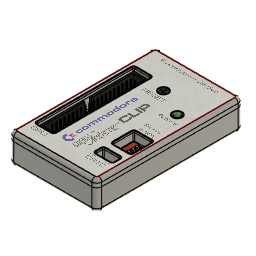
PETDiag_Clip_v3 v11 (Autodesk Fusion 360 design; units mm, degrees)
Autodesk Fusion 360 part; units mm, degrees
(part 1 of 3)
sketch "dxf" plane through (0, 0, 0) normal (0, 0, 1) x (1, 0, 0) in component "PCB"
  line L0 (47, 0) -> (47, 77)
  line L1 (0, 77) -> (0, 0)
  line L2 (0, 0) -> (47, 0)
  line L3 (47, 77) -> (0, 77)
  line L4 (1.7462, 63.1975) -> (1.7462, 63.3563)
  arc A0 (16.383, 5.334) -> (16.383, 7.366) centre (16.383, 6.35) ccw
  arc A1 (23.3363, 18.542) -> (20.7963, 18.542) centre (22.0663, 18.542) ccw
  circle A2 centre (5, 72) radius 3.1789
  line L5 (1.7462, 63.3563) -> (1.7462, 63.515)
  line L6 (1.7462, 40.8138) -> (1.7462, 62.0863)
  line L7 (1.7462, 63.6738) -> (1.7462, 67.96)
  line L8 (28.6703, 53.848) -> (15.4623, 53.848)
  line L9 (1.7462, 62.0863) -> (1.7462, 62.4038)
  line L10 (8.0963, 67.96) -> (9.525, 67.96)
  line L11 (1.7462, 63.515) -> (1.7462, 63.6738)
  line L12 (10.9538, 9.54) -> (9.525, 9.54)
  line L13 (23.3362, 18.542) -> (28.6703, 18.542)
  circle A3 centre (5, 5) radius 3.1789
  line L14 (15.4623, 18.542) -> (15.4623, 53.848)
  line L15 (1.7462, 67.96) -> (8.0963, 67.96)
  line L16 (16.383, 3.302) -> (35.687, 3.302)
  line L17 (1.7462, 62.88) -> (1.7462, 63.0388)
  line L18 (9.525, 9.54) -> (8.0963, 9.54)
  line L19 (1.7462, 62.7213) -> (1.7462, 62.88)
  line L20 (35.687, 9.398) -> (16.383, 9.398)
  line L21 (8.0963, 10.3337) -> (8.0963, 9.54)
  line L22 (2.54, 40.8138) -> (1.7462, 40.8138)
  line L23 (10.16, 67.1663) -> (10.16, 10.3337)
  line L24 (1.7462, 9.54) -> (1.7462, 36.6862)
  line L25 (3.0162, 10.81) -> (2.54, 10.3337)
  line L26 (28.6703, 18.542) -> (28.6703, 53.848)
  line L27 (7.366, 62.626) -> (7.874, 62.626)
  line L28 (8.0963, 10.3337) -> (2.54, 10.3337)
  line L29 (9.525, 66.69) -> (9.6838, 66.69)
  line L30 (9.525, 10.81) -> (8.0963, 10.81)
  line L31 (3.0162, 40.8138) -> (3.0162, 66.69)
  line L32 (1.7462, 36.6862) -> (1.7462, 40.8138)
  line L33 (8.0963, 66.69) -> (8.0963, 67.1663)
  arc A4 (10.9538, 38.2738) -> (10.9538, 39.385) centre (10.9538, 38.8294) ccw
  line L34 (15.4623, 18.542) -> (20.7963, 18.542)
  line L35 (1.7462, 62.5625) -> (1.7462, 62.7213)
  line L36 (1.7462, 63.1975) -> (1.7462, 63.0388)
  line L37 (2.54, 36.6862) -> (1.7462, 36.6862)
  line L38 (9.6838, 10.81) -> (9.525, 10.81)
  line L39 (8.0963, 9.54) -> (1.7462, 9.54)
  line L40 (3.0162, 36.6862) -> (2.54, 36.6862)
  line L41 (9.6838, 66.69) -> (9.6838, 10.81)
  line L42 (3.0162, 10.81) -> (3.0162, 36.6862)
  line L43 (1.7462, 62.5625) -> (1.7463, 62.5625)
  line L44 (8.0963, 10.81) -> (3.0162, 10.81)
  circle A5 centre (5, 5) radius 1.7463
  circle A6 centre (42, 72) radius 1.7463
  line L45 (35.687, 9.398) -> (35.687, 3.302)
  line L46 (9.525, 10.3337) -> (10.16, 10.3337)
  line L47 (16.383, 9.398) -> (16.383, 7.366)
  circle A7 centre (42, 5) radius 1.7463
  line L48 (4.826, 62.626) -> (5.334, 62.626)
  line L49 (9.525, 10.81) -> (9.525, 10.3337)
  line L50 (9.525, 66.69) -> (9.525, 67.1663)
  line L51 (16.383, 3.302) -> (16.383, 5.334)
  arc A8 (10.9538, 65.42) -> (10.9538, 66.69) centre (10.9538, 66.055) ccw
  line L52 (8.0963, 67.1663) -> (8.0963, 67.96)
  line L53 (9.525, 10.3337) -> (9.525, 9.54)
  line L54 (5.334, 62.626) -> (5.334, 63.134)
  line L55 (9.525, 67.1663) -> (9.525, 67.96)
  line L56 (3.0162, 66.69) -> (8.0963, 66.69)
  line L57 (10.16, 67.1663) -> (9.6838, 66.69)
  line L58 (1.7462, 62.4038) -> (1.7462, 62.5625)
  line L59 (10.9538, 67.96) -> (10.9538, 9.54)
  circle A9 centre (5, 72) radius 1.7463
  line L60 (2.2225, 62.7213) -> (2.2224, 62.7213)
  line L61 (10.16, 67.1663) -> (9.525, 67.1663)
  circle A10 centre (42, 72) radius 3.1789
  line L62 (2.54, 62.88) -> (2.5399, 62.88)
  line L63 (8.0963, 67.1663) -> (2.54, 67.1663)
  circle A11 centre (42, 5) radius 3.1789
  line L64 (5.334, 55.006) -> (5.334, 55.514)
  line L65 (7.366, 57.546) -> (7.874, 57.546)
  line L66 (7.366, 52.974) -> (7.366, 52.466)
  line L67 (7.874, 52.466) -> (7.874, 52.974)
  line L68 (4.826, 58.054) -> (4.826, 57.546)
  line L69 (5.334, 55.514) -> (4.826, 55.514)
  line L70 (5.334, 60.086) -> (5.334, 60.594)
  line L71 (4.826, 57.546) -> (5.334, 57.546)
  line L72 (7.874, 60.594) -> (7.366, 60.594)
  line L73 (4.826, 63.134) -> (4.826, 62.626)
  line L74 (7.874, 63.134) -> (7.366, 63.134)
  line L75 (7.366, 52.466) -> (7.874, 52.466)
  line L76 (7.874, 55.514) -> (7.366, 55.514)
  line L77 (4.826, 55.514) -> (4.826, 55.006)
  line L78 (4.826, 60.086) -> (5.334, 60.086)
  line L79 (2.54, 36.6862) -> (2.54, 10.3337)
  line L80 (4.826, 49.926) -> (5.334, 49.926)
  line L81 (7.874, 49.926) -> (7.874, 50.434)
  line L82 (4.826, 52.466) -> (5.334, 52.466)
  line L83 (7.366, 58.054) -> (7.366, 57.546)
  line L84 (7.874, 52.974) -> (7.366, 52.974)
  line L85 (3.0162, 36.6862) -> (3.0162, 40.8138)
  line L86 (9.6838, 10.81) -> (10.16, 10.3337)
  line L87 (5.334, 47.894) -> (4.826, 47.894)
  line L88 (7.366, 49.926) -> (7.874, 49.926)
  line L89 (9.525, 67.96) -> (10.9538, 67.96)
  line L90 (2.54, 62.88) -> (2.54, 67.1663)
  line L91 (7.366, 50.434) -> (7.366, 49.926)
  line L92 (5.334, 52.974) -> (4.826, 52.974)
  line L93 (7.366, 44.846) -> (7.874, 44.846)
  line L94 (7.874, 57.546) -> (7.874, 58.054)
  line L95 (2.54, 40.8138) -> (2.54, 62.88)
  line L96 (4.826, 60.594) -> (4.826, 60.086)
  line L97 (7.874, 55.006) -> (7.874, 55.514)
  line L98 (7.366, 55.514) -> (7.366, 55.006)
  line L99 (4.826, 50.434) -> (4.826, 49.926)
  line L100 (7.874, 50.434) -> (7.366, 50.434)
  line L101 (5.334, 50.434) -> (4.826, 50.434)
  line L102 (5.334, 58.054) -> (4.826, 58.054)
  line L103 (7.366, 45.354) -> (7.366, 44.846)
  arc A12 (10.9538, 10.81) -> (10.9538, 12.08) centre (10.9538, 11.445) ccw
  line L104 (5.334, 49.926) -> (5.334, 50.434)
  line L105 (4.826, 47.386) -> (5.334, 47.386)
  line L106 (5.334, 47.386) -> (5.334, 47.894)
  line L107 (4.826, 55.006) -> (5.334, 55.006)
  line L108 (7.366, 60.594) -> (7.366, 60.086)
  line L109 (3.0162, 40.8138) -> (2.54, 40.8138)
  line L110 (5.334, 63.134) -> (4.826, 63.134)
  line L111 (8.0963, 10.81) -> (8.0963, 10.3337)
  line L112 (7.874, 62.626) -> (7.874, 63.134)
  line L113 (2.54, 67.1663) -> (3.0162, 66.69)
  line L114 (8.0963, 66.69) -> (9.525, 66.69)
  line L115 (7.874, 60.086) -> (7.874, 60.594)
  line L116 (7.366, 63.134) -> (7.366, 62.626)
  line L117 (7.366, 47.386) -> (7.874, 47.386)
  line L118 (5.334, 60.594) -> (4.826, 60.594)
  line L119 (5.334, 52.466) -> (5.334, 52.974)
  line L120 (7.874, 47.894) -> (7.366, 47.894)
  line L121 (7.874, 47.386) -> (7.874, 47.894)
  line L122 (4.826, 47.894) -> (4.826, 47.386)
  line L123 (7.874, 58.054) -> (7.366, 58.054)
  line L124 (7.366, 34.686) -> (7.874, 34.686)
  line L125 (7.366, 32.654) -> (7.366, 32.146)
  line L126 (4.826, 32.654) -> (4.826, 32.146)
  line L127 (7.874, 32.654) -> (7.366, 32.654)
  line L128 (7.366, 47.894) -> (7.366, 47.386)
  line L129 (7.366, 37.734) -> (7.366, 37.226)
  line L130 (4.826, 39.766) -> (5.334, 39.766)
  line L131 (5.334, 45.354) -> (4.826, 45.354)
  line L132 (7.874, 40.274) -> (7.366, 40.274)
  line L133 (7.874, 30.114) -> (7.366, 30.114)
  line L134 (7.874, 42.306) -> (7.874, 42.814)
  line L135 (7.366, 60.086) -> (7.874, 60.086)
  line L136 (7.874, 42.814) -> (7.366, 42.814)
  line L137 (5.334, 32.654) -> (4.826, 32.654)
  line L138 (5.334, 37.734) -> (4.826, 37.734)
  line L139 (5.334, 42.814) -> (4.826, 42.814)
  line L140 (5.334, 40.274) -> (4.826, 40.274)
  line L141 (7.366, 55.006) -> (7.874, 55.006)
  line L142 (4.826, 42.814) -> (4.826, 42.306)
  line L143 (5.334, 42.306) -> (5.334, 42.814)
  line L144 (7.874, 44.846) -> (7.874, 45.354)
  line L145 (7.874, 32.146) -> (7.874, 32.654)
  line L146 (7.874, 45.354) -> (7.366, 45.354)
  line L147 (7.874, 34.686) -> (7.874, 35.194)
  line L148 (5.334, 39.766) -> (5.334, 40.274)
  line L149 (4.826, 44.846) -> (5.334, 44.846)
  line L150 (7.366, 35.194) -> (7.366, 34.686)
  line L151 (4.826, 40.274) -> (4.826, 39.766)
  line L152 (7.366, 32.146) -> (7.874, 32.146)
  line L153 (5.334, 25.034) -> (4.826, 25.034)
  line L154 (4.826, 19.446) -> (5.334, 19.446)
  line L155 (4.826, 32.146) -> (5.334, 32.146)
  line L156 (5.334, 29.606) -> (5.334, 30.114)
  line L157 (5.334, 19.954) -> (4.826, 19.954)
  line L158 (4.826, 25.034) -> (4.826, 24.526)
  line L159 (4.826, 34.686) -> (5.334, 34.686)
  line L160 (4.826, 35.194) -> (4.826, 34.686)
  line L161 (4.826, 37.226) -> (5.334, 37.226)
  line L162 (7.874, 37.226) -> (7.874, 37.734)
  line L163 (4.826, 45.354) -> (4.826, 44.846)
  line L164 (7.874, 29.606) -> (7.874, 30.114)
  line L165 (7.366, 37.226) -> (7.874, 37.226)
  line L166 (7.366, 42.306) -> (7.874, 42.306)
  line L167 (7.874, 39.766) -> (7.874, 40.274)
  line L168 (7.366, 29.606) -> (7.874, 29.606)
  line L169 (5.334, 37.226) -> (5.334, 37.734)
  line L170 (7.366, 40.274) -> (7.366, 39.766)
  line L171 (4.826, 19.954) -> (4.826, 19.446)
  line L172 (4.826, 21.986) -> (5.334, 21.986)
  line L173 (7.366, 30.114) -> (7.366, 29.606)
  line L174 (5.334, 27.574) -> (4.826, 27.574)
  line L175 (5.334, 57.546) -> (5.334, 58.054)
  line L176 (4.826, 52.974) -> (4.826, 52.466)
  line L177 (5.334, 32.146) -> (5.334, 32.654)
  line L178 (7.874, 35.194) -> (7.366, 35.194)
  line L179 (5.334, 44.846) -> (5.334, 45.354)
  line L180 (7.366, 39.766) -> (7.874, 39.766)
  line L181 (7.366, 42.814) -> (7.366, 42.306)
  line L182 (4.826, 37.734) -> (4.826, 37.226)
  line L183 (7.874, 37.734) -> (7.366, 37.734)
  line L184 (4.826, 30.114) -> (4.826, 29.606)
  line L185 (5.334, 34.686) -> (5.334, 35.194)
  line L186 (4.826, 42.306) -> (5.334, 42.306)
  line L187 (5.334, 35.194) -> (4.826, 35.194)
  line L188 (5.334, 22.494) -> (4.826, 22.494)
  line L189 (34.29, 53.975) -> (33.02, 53.975)
  line L190 (28.2575, 15.7163) -> (28.2575, 11.9063)
  line L191 (34.29, 48.895) -> (33.02, 48.895)
  line L192 (25.0825, 11.2713) -> (25.7175, 11.9063)
  line L193 (30.7975, 15.7163) -> (30.7975, 11.9063)
  line L194 (7.874, 19.954) -> (7.366, 19.954)
  line L195 (5.334, 21.986) -> (5.334, 22.494)
  line L196 (23.8125, 16.3513) -> (25.0825, 16.3513)
  line L197 (7.366, 25.034) -> (7.366, 24.526)
  line L198 (5.334, 19.446) -> (5.334, 19.954)
  line L199 (7.366, 16.906) -> (7.874, 16.906)
  line L200 (26.3525, 11.2713) -> (27.6225, 11.2713)
  line L201 (25.7175, 15.7163) -> (25.7175, 11.9063)
  line L202 (5.334, 16.906) -> (5.334, 17.414)
  line L203 (4.826, 17.414) -> (4.826, 16.906)
  line L204 (26.3525, 16.3513) -> (27.6225, 16.3513)
  line L205 (28.2575, 15.7163) -> (28.8925, 16.3513)
  line L206 (7.874, 24.526) -> (7.874, 25.034)
  line L207 (4.826, 14.874) -> (4.826, 14.366)
  line L208 (7.874, 19.446) -> (7.874, 19.954)
  line L209 (7.874, 25.034) -> (7.366, 25.034)
  line L210 (7.874, 27.066) -> (7.874, 27.574)
  line L211 (7.366, 27.574) -> (7.366, 27.066)
  line L212 (7.874, 27.574) -> (7.366, 27.574)
  line L213 (23.1775, 11.9063) -> (23.1775, 15.7163)
  line L214 (7.874, 14.874) -> (7.366, 14.874)
  line L215 (32.385, 52.07) -> (32.385, 53.975)
  line L216 (7.366, 19.446) -> (7.874, 19.446)
  line L217 (5.334, 30.114) -> (4.826, 30.114)
  line L218 (7.366, 19.954) -> (7.366, 19.446)
  line L219 (4.826, 16.906) -> (5.334, 16.906)
  line L220 (7.366, 21.986) -> (7.874, 21.986)
  line L221 (25.7175, 11.9063) -> (26.3525, 11.2713)
  line L222 (32.385, 49.53) -> (32.385, 50.8)
  line L223 (33.02, 53.975) -> (32.385, 53.975)
  line L224 (34.925, 50.8) -> (34.925, 49.53)
  line L225 (4.826, 22.494) -> (4.826, 21.986)
  line L226 (7.874, 14.366) -> (7.874, 14.874)
  line L227 (5.334, 14.366) -> (5.334, 14.874)
  line L228 (5.334, 27.066) -> (5.334, 27.574)
  line L229 (4.826, 27.066) -> (5.334, 27.066)
  line L230 (5.334, 14.874) -> (4.826, 14.874)
  line L231 (4.826, 27.574) -> (4.826, 27.066)
  line L232 (27.6225, 11.2713) -> (28.2575, 11.9063)
  line L233 (7.366, 14.874) -> (7.366, 14.366)
  line L234 (7.874, 17.414) -> (7.366, 17.414)
  line L235 (7.366, 22.494) -> (7.366, 21.986)
  line L236 (7.874, 22.494) -> (7.366, 22.494)
  line L237 (5.334, 17.414) -> (4.826, 17.414)
  line L238 (5.334, 24.526) -> (5.334, 25.034)
  line L239 (7.874, 21.986) -> (7.874, 22.494)
  line L240 (7.366, 24.526) -> (7.874, 24.526)
  line L241 (7.366, 27.066) -> (7.874, 27.066)
  line L242 (7.366, 17.414) -> (7.366, 16.906)
  line L243 (4.826, 24.526) -> (5.334, 24.526)
  line L244 (4.826, 14.366) -> (5.334, 14.366)
  line L245 (7.366, 14.366) -> (7.874, 14.366)
  line L246 (4.826, 29.606) -> (5.334, 29.606)
  line L247 (7.874, 16.906) -> (7.874, 17.414)
  line L248 (34.925, 52.07) -> (34.6075, 51.7525)
  line L249 (27.6225, 16.3513) -> (28.2575, 15.7163)
  line L250 (34.6075, 51.1175) -> (34.925, 50.8)
  line L251 (34.925, 53.34) -> (34.925, 52.07)
  circle A13 centre (23, 65) radius 1.75
  arc A14 (25.45, 63.25) -> (25.45, 62.45) centre (25.15, 62.85) ccw
  line L252 (34.925, 53.34) -> (34.29, 53.975)
  line L253 (25.7175, 15.7163) -> (26.3525, 16.3513)
  line L254 (32.7025, 51.7525) -> (32.385, 52.07)
  line L255 (30.1625, 11.2713) -> (30.7975, 11.9063)
  line L256 (45.7518, 33.9408) -> (42.4498, 33.9408)
  line L257 (26, 66.45) -> (26, 63.6)
  line L258 (23.1775, 11.9063) -> (23.1775, 11.2713)
  line L259 (30.1625, 16.3513) -> (30.7975, 15.7163)
  line L260 (25.0825, 16.3513) -> (25.7175, 15.7163)
  line L261 (28.8925, 16.3513) -> (30.1625, 16.3513)
  line L262 (32.385, 50.8) -> (32.7025, 51.1175)
  line L263 (23.1775, 11.2713) -> (25.0825, 11.2713)
  line L264 (28.8925, 11.2713) -> (30.1625, 11.2713)
  arc A15 (20.55, 62.45) -> (20.5, 63.2) centre (20.8502, 62.8467) ccw
  circle A16 centre (23, 65) radius 1.4
  line L265 (28.2575, 11.9063) -> (28.8925, 11.2713)
  line L266 (23.1775, 15.7163) -> (23.8125, 16.3513)
  line L267 (25.4, 62) -> (20.25, 62)
  line L268 (20, 63.55) -> (20, 66.45)
  arc A17 (20.55, 66.75) -> (20.5, 67.5) centre (20.8502, 67.1467) ccw
  line L269 (33.02, 48.895) -> (32.385, 49.53)
  line L270 (34.925, 49.53) -> (34.29, 48.895)
  line L271 (39.1478, 33.4327) -> (42.4498, 33.4327)
  line L272 (20.25, 68) -> (25.75, 68)
  line L273 (41.6878, 32.6707) -> (38.8938, 32.6707)
  line L274 (39.1478, 33.9408) -> (35.8458, 33.9408)
  line L275 (42.4498, 32.6707) -> (42.7037, 32.6707)
  line L276 (38.8938, 23.5267) -> (41.6878, 23.5267)
  line L277 (41.6878, 25.0508) -> (38.8938, 25.0508)
  line L278 (38.8938, 23.5267) -> (38.8938, 25.0508)
  line L279 (42.7037, 31.1468) -> (42.4498, 31.1468)
  line L280 (40.7988, 24.7968) -> (39.1478, 24.7968)
  line L281 (42.7037, 28.8608) -> (42.7037, 28.6068)
  line L282 (42.7037, 23.5267) -> (42.4498, 23.5267)
  line L283 (42.7037, 25.0508) -> (42.7037, 24.7968)
  line L284 (40.7988, 29.8768) -> (39.1478, 29.8768)
  line L285 (42.4498, 30.1308) -> (42.7037, 30.1308)
  line L286 (38.8938, 31.1468) -> (41.6878, 31.1468)
  line L287 (40.7988, 26.3208) -> (39.1478, 26.3208)
  line L288 (42.4498, 33.4327) -> (42.4498, 33.9408)
  line L289 (42.7037, 31.4008) -> (42.7037, 31.1468)
  line L290 (38.8938, 28.6068) -> (38.8938, 30.1308)
  line L291 (42.7037, 26.3208) -> (42.7037, 26.0668)
  line L292 (40.7988, 28.8608) -> (39.1478, 28.8608)
  line L293 (40.7988, 27.3368) -> (39.1478, 27.3368)
  line L294 (39.1478, 29.8768) -> (39.1478, 28.8608)
  line L295 (41.6878, 30.1308) -> (38.8938, 30.1308)
  line L296 (38.8938, 28.6068) -> (41.6878, 28.6068)
  line L297 (39.1478, 33.9408) -> (39.1478, 33.4327)
  line L298 (42.7037, 27.5907) -> (42.7037, 27.3368)
  line L299 (38.8938, 26.0668) -> (38.8938, 27.5907)
  line L300 (42.7037, 30.1308) -> (42.7037, 29.8768)
  arc A18 (25.45, 67.55) -> (25.5, 66.8) centre (25.1498, 67.1533) ccw
  line L301 (42.7037, 32.6707) -> (42.7037, 32.4168)
  line L302 (40.7988, 32.4168) -> (39.1478, 32.4168)
  line L303 (42.4498, 27.5907) -> (42.7037, 27.5907)
  line L304 (42.7037, 23.7808) -> (42.7037, 23.5267)
  line L305 (40.7988, 31.4008) -> (39.1478, 31.4008)
  line L306 (41.6878, 27.5907) -> (38.8938, 27.5907)
  line L307 (38.8938, 31.1468) -> (38.8938, 32.6707)
  line L308 (42.4498, 25.0508) -> (42.7037, 25.0508)
  line L309 (42.7037, 28.6068) -> (42.4498, 28.6068)
  line L310 (38.8938, 26.0668) -> (41.6878, 26.0668)
  line L311 (42.4498, 33.9408) -> (39.1478, 33.9408)
  line L312 (42.7037, 26.0668) -> (42.4498, 26.0668)
  line L313 (40.7988, 23.7808) -> (39.1478, 23.7808)
  line L314 (39.7828, 27.3368) -> (39.7828, 26.3208)
  line L315 (40.7988, 28.8608) -> (40.7988, 29.8768)
  line L316 (40.7988, 31.4008) -> (40.7988, 32.4168)
  line L317 (39.5288, 32.4168) -> (39.1478, 32.4168)
  line L318 (39.1478, 26.3208) -> (39.5288, 26.3208)
  line L319 (40.4178, 23.7808) -> (40.7988, 23.7808)
  line L320 (39.1478, 23.7808) -> (39.5288, 23.7808)
  line L321 (39.7828, 32.4168) -> (39.7828, 31.4008)
  line L322 (40.4178, 24.7968) -> (40.4178, 23.7808)
  line L323 (39.5288, 23.7808) -> (39.5288, 24.7968)
  line L324 (39.1478, 31.4008) -> (39.5288, 31.4008)
  line L325 (39.5288, 26.3208) -> (39.5288, 27.3368)
  line L326 (39.7828, 26.3208) -> (40.1638, 26.3208)
  line L327 (40.1638, 23.7808) -> (40.1638, 24.7968)
  line L328 (40.4178, 28.8608) -> (40.7988, 28.8608)
  line L329 (40.1638, 27.3368) -> (39.7828, 27.3368)
  line L330 (39.7828, 23.7808) -> (40.1638, 23.7808)
  line L331 (39.7828, 28.8608) -> (40.1638, 28.8608)
  line L332 (39.1478, 24.7968) -> (39.1478, 23.7808)
  line L333 (40.4178, 29.8768) -> (40.4178, 28.8608)
  line L334 (40.7988, 32.4168) -> (40.4178, 32.4168)
  line L335 (39.5288, 31.4008) -> (39.5288, 32.4168)
  line L336 (40.7988, 23.7808) -> (40.7988, 24.7968)
  line L337 (40.1638, 29.8768) -> (39.7828, 29.8768)
  line L338 (40.7988, 26.3208) -> (40.7988, 27.3368)
  line L339 (39.7828, 31.4008) -> (40.1638, 31.4008)
  line L340 (40.4178, 32.4168) -> (40.4178, 31.4008)
  line L341 (40.1638, 31.4008) -> (40.1638, 32.4168)
  line L342 (40.4178, 31.4008) -> (40.7988, 31.4008)
  line L343 (40.1638, 32.4168) -> (39.7828, 32.4168)
  line L344 (40.7988, 27.3368) -> (40.4178, 27.3368)
  line L345 (39.7828, 29.8768) -> (39.7828, 28.8608)
  line L346 (39.5288, 28.8608) -> (39.5288, 29.8768)
  line L347 (39.1478, 27.3368) -> (39.1478, 26.3208)
  line L348 (39.1478, 28.8608) -> (39.5288, 28.8608)
  line L349 (40.1638, 28.8608) -> (40.1638, 29.8768)
  line L350 (39.5288, 24.7968) -> (39.1478, 24.7968)
  line L351 (39.5288, 27.3368) -> (39.1478, 27.3368)
  line L352 (39.1478, 32.4168) -> (39.1478, 31.4008)
  line L353 (40.7988, 29.8768) -> (40.4178, 29.8768)
  line L354 (40.4178, 26.3208) -> (40.7988, 26.3208)
  line L355 (40.4178, 27.3368) -> (40.4178, 26.3208)
  line L356 (40.7988, 24.7968) -> (40.4178, 24.7968)
  line L357 (39.7828, 24.7968) -> (39.7828, 23.7808)
  line L358 (40.1638, 26.3208) -> (40.1638, 27.3368)
  line L359 (40.1638, 24.7968) -> (39.7828, 24.7968)
  line L360 (39.5288, 29.8768) -> (39.1478, 29.8768)
  line L361 (24.7015, 12.2872) -> (24.7015, 12.7952)
  line L362 (24.7015, 12.7952) -> (24.1935, 12.7952)
  line L363 (33.401, 52.959) -> (33.401, 52.451)
  line L364 (34.6075, 51.7525) -> (34.29, 51.435)
  line L365 (34.29, 51.435) -> (33.02, 51.435)
  line L366 (24.1935, 12.7952) -> (24.1935, 12.2872)
  line L367 (33.909, 52.451) -> (33.909, 52.959)
  line L368 (24.7015, 14.8273) -> (24.7015, 15.3353)
  line L369 (26.7335, 12.2872) -> (27.2415, 12.2872)
  line L370 (29.2735, 15.3353) -> (29.2735, 14.8273)
  line L371 (33.909, 52.959) -> (33.401, 52.959)
  line L372 (26.7335, 12.7952) -> (26.7335, 12.2872)
  line L373 (29.7815, 12.2872) -> (29.7815, 12.7952)
  line L374 (32.7025, 51.1175) -> (33.02, 51.435)
  line L375 (33.401, 50.419) -> (33.401, 49.911)
  line L376 (33.909, 50.419) -> (33.401, 50.419)
  line L377 (33.02, 51.435) -> (32.7025, 51.7525)
  line L378 (34.29, 51.435) -> (34.6075, 51.1175)
  line L379 (33.401, 52.451) -> (33.909, 52.451)
  line L380 (33.909, 49.911) -> (33.909, 50.419)
  line L381 (33.401, 49.911) -> (33.909, 49.911)
  line L382 (24.1935, 12.2872) -> (24.7015, 12.2872)
  line L383 (27.2415, 14.8273) -> (27.2415, 15.3353)
  line L384 (25.75, 68) -> (25.8, 68)
  line L385 (20, 63.1) -> (19.5, 63.1)
  line L386 (19.5, 63.1) -> (19.5, 62.4)
  line L387 (26.5, 63.1) -> (26, 63.1)
  arc A19 (25.5, 66.8) -> (25.45, 67.55) centre (25.1498, 67.1533) ccw
  line L388 (26, 67.8) -> (26, 66.45)
  line L389 (26, 63.1) -> (26, 62.4)
  arc A20 (25.45, 62.45) -> (25.45, 63.25) centre (25.15, 62.85) ccw
  line L390 (26, 67.6) -> (26, 66.9)
  line L391 (20, 62.2) -> (20, 63.55)
  line L392 (25.8, 62) -> (25.4, 62)
  line L393 (26, 66.9) -> (26.5, 66.9)
  arc A21 (20.5, 63.2) -> (20.55, 62.45) centre (20.8502, 62.8467) ccw
  arc A22 (20.2, 68) -> (20, 67.8) centre (20.2, 67.8) ccw
  arc A23 (20, 62.2) -> (20.2, 62) centre (20.2, 62.2) ccw
  line L394 (29.7815, 12.7952) -> (29.2735, 12.7952)
  line L395 (19.5, 66.9) -> (20, 66.9)
  line L396 (26, 62.4) -> (26.5, 62.4)
  line L397 (26.5, 62.4) -> (26.5, 63.1)
  arc A24 (20.5, 67.5) -> (20.55, 66.75) centre (20.8502, 67.1467) ccw
  line L398 (27.2415, 12.2872) -> (27.2415, 12.7952)
  line L399 (24.7015, 15.3353) -> (24.1935, 15.3353)
  line L400 (19.5, 62.4) -> (20, 62.4)
  line L401 (42.7037, 27.3368) -> (42.7037, 26.3208)
  line L402 (29.2735, 14.8273) -> (29.7815, 14.8273)
  line L403 (42.4498, 28.6068) -> (41.6878, 28.6068)
  line L404 (20, 66.9) -> (20, 67.6)
  line L405 (42.7037, 24.7968) -> (42.7037, 23.7808)
  line L406 (20.25, 62) -> (20.2, 62)
  line L407 (42.4498, 30.1308) -> (41.6878, 30.1308)
  line L408 (20, 66.45) -> (20, 67.8)
  line L409 (26.5, 67.6) -> (26, 67.6)
  line L410 (42.4498, 31.1468) -> (41.6878, 31.1468)
  line L411 (19.5, 67.6) -> (19.5, 66.9)
  line L412 (42.4498, 23.5267) -> (41.6878, 23.5267)
  line L413 (42.4498, 27.5907) -> (41.6878, 27.5907)
  line L414 (27.2415, 12.7952) -> (26.7335, 12.7952)
  line L415 (29.7815, 14.8273) -> (29.7815, 15.3353)
  line L416 (26.7335, 15.3353) -> (26.7335, 14.8273)
  line L417 (29.2735, 12.7952) -> (29.2735, 12.2872)
  line L418 (20, 62.4) -> (20, 63.1)
  line L419 (20, 67.6) -> (19.5, 67.6)
  line L420 (26, 63.6) -> (26, 62.2)
  arc A25 (25.8, 62) -> (26, 62.2) centre (25.8, 62.2) ccw
  line L421 (24.1935, 15.3353) -> (24.1935, 14.8273)
  line L422 (26.7335, 14.8273) -> (27.2415, 14.8273)
  line L423 (29.2735, 12.2872) -> (29.7815, 12.2872)
  line L424 (27.2415, 15.3353) -> (26.7335, 15.3353)
  line L425 (29.7815, 15.3353) -> (29.2735, 15.3353)
  line L426 (20.2, 68) -> (20.25, 68)
  line L427 (26.5, 66.9) -> (26.5, 67.6)
  line L428 (24.1935, 14.8273) -> (24.7015, 14.8273)
  arc A26 (26, 67.8) -> (25.8, 68) centre (25.8, 67.8) ccw
  line L429 (37.7578, 23.9571) -> (37.7578, 24.7333)
  line L430 (37.4474, 24.5004) -> (38.0682, 24.5004)
  line L431 (38.0682, 29.0371) -> (38.0682, 29.8133)
  line L432 (43.7903, 31.7008) -> (44.4112, 31.7008)
  line L433 (42.4498, 25.0508) -> (41.6878, 25.0508)
  line L434 (36.9817, 31.3231) -> (36.6713, 31.7112)
  arc A27 (37.2921, 29.6968) -> (37.0205, 29.8132) centre (37.0205, 29.4381) ccw
  line L435 (37.2921, 26.9628) -> (37.2921, 26.6524)
  line L436 (36.6713, 24.2676) -> (37.7578, 23.9571)
  line L437 (43.4023, 32.3391) -> (44.7993, 33.1153)
  line L438 (42.4498, 26.0668) -> (41.6878, 26.0668)
  line L439 (42.7037, 29.8768) -> (42.7037, 28.8608)
  line L440 (38.0682, 31.3231) -> (38.0682, 32.0993)
  line L441 (38.0682, 26.4971) -> (38.0682, 26.8852)
  line L442 (42.4498, 32.6707) -> (41.6878, 32.6707)
  arc A28 (37.2921, 26.9628) -> (36.6713, 26.9628) centre (36.9817, 26.9628) ccw
  arc A29 (44.4112, 30.9246) -> (44.4112, 31.7008) centre (44.4112, 31.3127) ccw
  line L443 (44.4112, 30.9247) -> (43.7903, 30.9247)
  line L444 (36.6713, 26.4971) -> (36.6713, 26.9628)
  line L445 (37.2921, 29.6968) -> (38.0682, 29.0371)
  line L446 (44.7993, 33.1153) -> (43.4023, 33.1153)
  line L447 (42.7037, 32.4168) -> (42.7037, 31.4008)
  arc A30 (38.0683, 26.8852) -> (37.2921, 26.8852) centre (37.6802, 26.8852) ccw
  arc A31 (37.0205, 29.8133) -> (36.6712, 29.464) centre (37.0205, 29.464) ccw
  line L448 (44.7993, 32.3391) -> (43.4023, 32.3391)
  line L449 (36.6713, 31.7112) -> (38.0682, 31.7112)
  arc A32 (36.6712, 29.464) -> (36.9817, 29.0371) centre (37.1199, 29.464) ccw
  arc A33 (43.7903, 31.7008) -> (43.7903, 30.9246) centre (43.7903, 31.3127) ccw
  line L450 (47, 0) -> (47, 77)
  line L451 (0, 77) -> (0, 0)
  line L452 (0, 0) -> (47, 0)
  line L453 (47, 77) -> (0, 77)
  line L454 (13.1763, 15.0813) -> (18.2563, 15.0813)
  line L455 (13.1763, 15.0813) -> (13.1763, 12.5412)
  line L456 (13.335, 6.35) -> (13.335, 11.43)
  line L457 (15.875, 11.43) -> (15.875, 6.35)
  line L458 (18.2563, 12.5412) -> (18.2563, 15.0813)
  line L459 (15.875, 11.43) -> (13.335, 11.43)
  line L460 (18.2563, 12.5412) -> (13.1763, 12.5412)
  line L461 (12.2813, 69.2525) -> (17.8813, 69.2525)
  arc A34 (16.383, 5.334) -> (16.383, 7.366) centre (16.383, 6.35) ccw
  line L462 (12.2813, 61.4525) -> (12.2813, 60.4525)
  circle A35 centre (42, 5) radius 1.7463
  circle A36 centre (42, 72) radius 3.1789
  line L463 (17.8813, 59.6525) -> (12.2813, 59.6525)
  line L464 (16.383, 3.302) -> (35.687, 3.302)
  line L465 (14.5813, 59.6525) -> (14.5813, 58.0525)
  circle A37 centre (5, 72) radius 1.7463
  line L466 (15.4623, 18.542) -> (15.4623, 53.848)
  line L467 (35.687, 9.398) -> (35.687, 3.302)
  line L468 (8.0963, 9.54) -> (1.7462, 9.54)
  circle A38 centre (5, 5) radius 3.1789
  line L469 (1.7462, 9.54) -> (1.7462, 36.6862)
  line L470 (15.4623, 18.542) -> (20.7963, 18.542)
  line L471 (15.5813, 58.0525) -> (15.5813, 59.6525)
  line L472 (15.5813, 59.6525) -> (14.5813, 59.6525)
  line L473 (1.7462, 36.6862) -> (1.7462, 40.8138)
  line L474 (28.6703, 53.848) -> (15.4623, 53.848)
  line L475 (16.383, 9.398) -> (16.383, 7.366)
  line L476 (1.7462, 40.8138) -> (1.7462, 62.0863)
  line L477 (9.525, 9.54) -> (8.0963, 9.54)
  line L478 (14.5813, 69.2525) -> (15.5813, 69.2525)
  line L479 (12.2813, 59.6525) -> (12.2813, 69.2525)
  line L480 (14.5813, 58.0525) -> (15.5813, 58.0525)
  line L481 (28.6703, 18.542) -> (28.6703, 53.848)
  line L482 (1.7462, 62.0863) -> (1.7462, 62.4038)
  line L483 (17.8813, 60.4525) -> (17.8813, 61.4525)
  line L484 (1.7462, 63.515) -> (1.7462, 63.6738)
  line L485 (10.9538, 67.96) -> (10.9538, 9.54)
  line L486 (10.9538, 9.54) -> (9.525, 9.54)
  circle A39 centre (5, 5) radius 1.7463
  line L487 (1.7462, 63.3563) -> (1.7462, 63.515)
  line L488 (17.8813, 69.2525) -> (17.8813, 59.6525)
  line L489 (14.5813, 70.8525) -> (14.5813, 69.2525)
  line L490 (35.687, 9.398) -> (16.383, 9.398)
  line L491 (15.5813, 70.8525) -> (14.5813, 70.8525)
  line L492 (13.335, 6.35) -> (15.875, 6.35)
  line L493 (16.383, 3.302) -> (16.383, 5.334)
  line L494 (23.3362, 18.542) -> (28.6703, 18.542)
  line L495 (1.7462, 63.1975) -> (1.7462, 63.3563)
  circle A40 centre (5, 72) radius 3.1789
  line L496 (15.5813, 69.2525) -> (15.5813, 70.8525)
  circle A41 centre (42, 72) radius 1.7463
  line L497 (1.7462, 62.4038) -> (1.7462, 62.5625)
  line L498 (9.525, 67.1663) -> (9.525, 67.96)
  line L499 (8.0963, 10.81) -> (3.0162, 10.81)
  line L500 (2.2224, 62.7213) -> (1.7462, 63.1975)
  line L501 (3.0162, 36.6862) -> (3.0162, 40.8138)
  line L502 (8.0963, 66.69) -> (8.0963, 67.1663)
  circle A42 centre (42, 5) radius 3.1789
  line L503 (9.525, 66.69) -> (9.525, 67.1663)
  line L504 (8.0963, 10.3337) -> (2.54, 10.3337)
  line L505 (3.0162, 10.81) -> (2.54, 10.3337)
  line L506 (9.525, 67.96) -> (10.9538, 67.96)
  line L507 (8.0963, 66.69) -> (9.525, 66.69)
  arc A43 (10.9538, 38.2738) -> (10.9538, 39.385) centre (10.9538, 38.8294) ccw
  line L508 (3.0162, 36.6862) -> (2.54, 36.6862)
  line L509 (1.7462, 62.88) -> (1.7462, 63.0388)
  line L510 (10.16, 67.1663) -> (10.16, 10.3337)
  line L511 (12.2813, 60.4525) -> (17.8813, 60.4525)
  line L512 (8.0963, 67.96) -> (9.525, 67.96)
  line L513 (2.3812, 62.7213) -> (2.0637, 62.4038)
  arc A44 (23.3363, 18.542) -> (20.7963, 18.542) centre (22.0663, 18.542) ccw
  line L514 (2.54, 40.8138) -> (1.7462, 40.8138)
  line L515 (1.7462, 63.1975) -> (1.7462, 63.0388)
  line L516 (3.0162, 66.69) -> (8.0963, 66.69)
  line L517 (8.0963, 67.1663) -> (8.0963, 67.96)
  arc A45 (10.9538, 65.42) -> (10.9538, 66.69) centre (10.9538, 66.055) ccw
  line L518 (3.0162, 40.8138) -> (2.54, 40.8138)
  line L519 (9.525, 66.69) -> (9.6838, 66.69)
  line L520 (1.7462, 67.96) -> (8.0963, 67.96)
  line L521 (10.16, 67.1663) -> (9.6838, 66.69)
  line L522 (2.54, 40.8138) -> (2.54, 62.88)
  line L523 (9.6838, 10.81) -> (9.525, 10.81)
  line L524 (1.7462, 63.6738) -> (1.7462, 67.96)
  line L525 (2.5399, 62.88) -> (2.3812, 62.7213)
  line L526 (2.54, 36.6862) -> (1.7462, 36.6862)
  line L527 (8.0963, 67.1663) -> (2.54, 67.1663)
  line L528 (9.525, 10.3337) -> (9.525, 9.54)
  line L529 (1.7462, 63.0388) -> (2.2225, 62.5625)
  line L530 (2.54, 62.88) -> (1.7462, 63.6738)
  line L531 (8.0963, 10.3337) -> (8.0963, 9.54)
  line L532 (9.6838, 10.81) -> (10.16, 10.3337)
  line L533 (10.16, 67.1663) -> (9.525, 67.1663)
  arc A46 (10.9538, 10.81) -> (10.9538, 12.08) centre (10.9538, 11.445) ccw
  line L534 (1.7462, 62.88) -> (2.0637, 62.5625)
  line L535 (2.54, 67.1663) -> (3.0162, 66.69)
  line L536 (9.525, 10.81) -> (8.0963, 10.81)
  line L537 (17.8813, 61.4525) -> (12.2813, 61.4525)
  line L538 (1.7462, 62.5625) -> (1.7463, 62.5625)
  line L539 (3.0162, 40.8138) -> (3.0162, 66.69)
  line L540 (9.525, 10.81) -> (9.525, 10.3337)
  line L541 (1.7462, 62.5625) -> (1.7462, 62.7213)
  line L542 (1.7462, 62.7213) -> (1.7462, 62.88)
  line L543 (3.0162, 10.81) -> (3.0162, 36.6862)
  line L544 (8.0963, 10.81) -> (8.0963, 10.3337)
  line L545 (7.874, 52.466) -> (7.874, 52.974)
  line L546 (5.334, 63.134) -> (4.826, 63.134)
  line L547 (2.3812, 62.88) -> (1.7462, 63.515)
  line L548 (5.334, 60.086) -> (5.334, 60.594)
  line L549 (7.366, 63.134) -> (7.366, 62.626)
  line L550 (7.874, 55.514) -> (7.366, 55.514)
  line L551 (4.826, 60.086) -> (5.334, 60.086)
  line L552 (9.525, 10.3337) -> (10.16, 10.3337)
  line L553 (7.366, 52.466) -> (7.874, 52.466)
  line L554 (5.334, 55.006) -> (5.334, 55.514)
  line L555 (2.54, 36.6862) -> (2.54, 10.3337)
  line L556 (7.874, 58.054) -> (7.366, 58.054)
  line L557 (7.366, 55.514) -> (7.366, 55.006)
  line L558 (4.826, 57.546) -> (5.334, 57.546)
  line L559 (7.874, 49.926) -> (7.874, 50.434)
  line L560 (7.366, 55.006) -> (7.874, 55.006)
  line L561 (1.7462, 63.3563) -> (2.3812, 62.7213)
  line L562 (1.7462, 62.4038) -> (1.905, 62.245)
  line L563 (4.826, 63.134) -> (4.826, 62.626)
  line L564 (4.826, 50.434) -> (4.826, 49.926)
  line L565 (7.874, 60.594) -> (7.366, 60.594)
  line L566 (34.925, 53.34) -> (34.925, 52.07)
  line L567 (4.826, 52.974) -> (4.826, 52.466)
  line L568 (7.366, 60.086) -> (7.874, 60.086)
  line L569 (4.826, 60.594) -> (4.826, 60.086)
  line L570 (7.366, 62.626) -> (7.874, 62.626)
  line L571 (1.7463, 62.5625) -> (1.905, 62.4038)
  line L572 (7.874, 60.086) -> (7.874, 60.594)
  line L573 (7.366, 52.974) -> (7.366, 52.466)
  line L574 (2.2225, 62.7213) -> (2.2224, 62.7213)
  line L575 (9.6838, 66.69) -> (9.6838, 10.81)
  line L576 (5.334, 52.974) -> (4.826, 52.974)
  line L577 (7.874, 50.434) -> (7.366, 50.434)
  line L578 (2.0637, 62.4038) -> (1.7462, 62.0863)
  line L579 (7.366, 57.546) -> (7.874, 57.546)
  line L580 (7.366, 49.926) -> (7.874, 49.926)
  line L581 (4.826, 62.626) -> (5.334, 62.626)
  line L582 (1.7462, 62.7213) -> (2.0637, 62.4038)
  line L583 (5.334, 62.626) -> (5.334, 63.134)
  line L584 (2.54, 62.88) -> (2.5399, 62.88)
  line L585 (7.874, 55.006) -> (7.874, 55.514)
  line L586 (7.366, 58.054) -> (7.366, 57.546)
  line L587 (4.826, 58.054) -> (4.826, 57.546)
  line L588 (5.334, 60.594) -> (4.826, 60.594)
  line L589 (5.334, 58.054) -> (4.826, 58.054)
  line L590 (7.874, 63.134) -> (7.366, 63.134)
  line L591 (7.366, 60.594) -> (7.366, 60.086)
  line L592 (4.826, 49.926) -> (5.334, 49.926)
  line L593 (4.826, 55.514) -> (4.826, 55.006)
  line L594 (5.334, 52.466) -> (5.334, 52.974)
  line L595 (5.334, 49.926) -> (5.334, 50.434)
  line L596 (7.874, 57.546) -> (7.874, 58.054)
  line L597 (2.54, 62.88) -> (2.54, 67.1663)
  line L598 (5.334, 47.894) -> (4.826, 47.894)
  line L599 (7.874, 47.386) -> (7.874, 47.894)
  line L600 (4.826, 37.734) -> (4.826, 37.226)
  line L601 (7.366, 47.386) -> (7.874, 47.386)
  line L602 (7.874, 37.226) -> (7.874, 37.734)
  line L603 (4.826, 37.226) -> (5.334, 37.226)
  line L604 (7.874, 44.846) -> (7.874, 45.354)
  line L605 (7.366, 42.814) -> (7.366, 42.306)
  line L606 (7.874, 35.194) -> (7.366, 35.194)
  line L607 (5.334, 45.354) -> (4.826, 45.354)
  line L608 (7.874, 52.974) -> (7.366, 52.974)
  line L609 (7.874, 47.894) -> (7.366, 47.894)
  line L610 (7.874, 40.274) -> (7.366, 40.274)
  line L611 (7.366, 37.226) -> (7.874, 37.226)
  line L612 (5.334, 50.434) -> (4.826, 50.434)
  line L613 (4.826, 52.466) -> (5.334, 52.466)
  line L614 (5.334, 42.306) -> (5.334, 42.814)
  line L615 (5.334, 47.386) -> (5.334, 47.894)
  line L616 (5.334, 34.686) -> (5.334, 35.194)
  line L617 (7.366, 45.354) -> (7.366, 44.846)
  line L618 (4.826, 42.306) -> (5.334, 42.306)
  line L619 (7.874, 45.354) -> (7.366, 45.354)
  line L620 (7.874, 62.626) -> (7.874, 63.134)
  line L621 (4.826, 47.894) -> (4.826, 47.386)
  line L622 (4.826, 47.386) -> (5.334, 47.386)
  line L623 (7.366, 35.194) -> (7.366, 34.686)
  line L624 (4.826, 44.846) -> (5.334, 44.846)
  line L625 (7.366, 44.846) -> (7.874, 44.846)
  line L626 (7.874, 42.814) -> (7.366, 42.814)
  line L627 (5.334, 40.274) -> (4.826, 40.274)
  line L628 (4.826, 35.194) -> (4.826, 34.686)
  line L629 (5.334, 55.514) -> (4.826, 55.514)
  line L630 (7.874, 42.306) -> (7.874, 42.814)
  line L631 (7.366, 47.894) -> (7.366, 47.386)
  line L632 (4.826, 45.354) -> (4.826, 44.846)
  line L633 (7.366, 40.274) -> (7.366, 39.766)
  line L634 (7.366, 50.434) -> (7.366, 49.926)
  line L635 (4.826, 55.006) -> (5.334, 55.006)
  line L636 (7.366, 37.734) -> (7.366, 37.226)
  line L637 (5.334, 57.546) -> (5.334, 58.054)
  line L638 (7.366, 32.146) -> (7.874, 32.146)
  line L639 (4.826, 32.654) -> (4.826, 32.146)
  line L640 (4.826, 40.274) -> (4.826, 39.766)
  line L641 (4.826, 39.766) -> (5.334, 39.766)
  line L642 (7.874, 32.146) -> (7.874, 32.654)
  line L643 (5.334, 37.734) -> (4.826, 37.734)
  line L644 (7.366, 42.306) -> (7.874, 42.306)
  line L645 (5.334, 42.814) -> (4.826, 42.814)
  line L646 (7.874, 37.734) -> (7.366, 37.734)
  line L647 (7.366, 29.606) -> (7.874, 29.606)
  line L648 (5.334, 44.846) -> (5.334, 45.354)
  line L649 (5.334, 35.194) -> (4.826, 35.194)
  line L650 (4.826, 42.814) -> (4.826, 42.306)
  line L651 (7.366, 34.686) -> (7.874, 34.686)
  line L652 (5.334, 32.654) -> (4.826, 32.654)
  line L653 (7.874, 39.766) -> (7.874, 40.274)
  line L654 (7.874, 32.654) -> (7.366, 32.654)
  line L655 (7.366, 39.766) -> (7.874, 39.766)
  line L656 (5.334, 39.766) -> (5.334, 40.274)
  line L657 (7.874, 34.686) -> (7.874, 35.194)
  line L658 (7.366, 30.114) -> (7.366, 29.606)
  line L659 (4.826, 32.146) -> (5.334, 32.146)
  line L660 (5.334, 32.146) -> (5.334, 32.654)
  line L661 (5.334, 37.226) -> (5.334, 37.734)
  line L662 (4.826, 34.686) -> (5.334, 34.686)
  line L663 (7.366, 32.654) -> (7.366, 32.146)
  line L664 (4.826, 16.906) -> (5.334, 16.906)
  line L665 (4.826, 29.606) -> (5.334, 29.606)
  line L666 (7.874, 27.574) -> (7.366, 27.574)
  line L667 (4.826, 19.446) -> (5.334, 19.446)
  line L668 (4.826, 21.986) -> (5.334, 21.986)
  line L669 (7.874, 14.366) -> (7.874, 14.874)
  line L670 (7.874, 27.066) -> (7.874, 27.574)
  line L671 (5.334, 30.114) -> (4.826, 30.114)
  line L672 (5.334, 17.414) -> (4.826, 17.414)
  line L673 (4.826, 14.874) -> (4.826, 14.366)
  line L674 (7.874, 25.034) -> (7.366, 25.034)
  line L675 (5.334, 16.906) -> (5.334, 17.414)
  line L676 (7.366, 19.446) -> (7.874, 19.446)
  line L677 (7.366, 21.986) -> (7.874, 21.986)
  line L678 (7.874, 19.446) -> (7.874, 19.954)
  line L679 (7.874, 30.114) -> (7.366, 30.114)
  line L680 (5.334, 19.954) -> (4.826, 19.954)
  line L681 (7.874, 29.606) -> (7.874, 30.114)
  line L682 (7.874, 24.526) -> (7.874, 25.034)
  line L683 (4.826, 14.366) -> (5.334, 14.366)
  line L684 (7.874, 19.954) -> (7.366, 19.954)
  line L685 (4.826, 22.494) -> (4.826, 21.986)
  line L686 (4.826, 30.114) -> (4.826, 29.606)
  line L687 (7.366, 22.494) -> (7.366, 21.986)
  line L688 (5.334, 25.034) -> (4.826, 25.034)
  line L689 (5.334, 22.494) -> (4.826, 22.494)
  line L690 (7.366, 27.574) -> (7.366, 27.066)
  line L691 (4.826, 27.066) -> (5.334, 27.066)
  line L692 (4.826, 27.574) -> (4.826, 27.066)
  line L693 (5.334, 27.066) -> (5.334, 27.574)
  line L694 (7.366, 27.066) -> (7.874, 27.066)
  line L695 (7.874, 21.986) -> (7.874, 22.494)
  line L696 (4.826, 25.034) -> (4.826, 24.526)
  line L697 (5.334, 21.986) -> (5.334, 22.494)
  line L698 (4.826, 19.954) -> (4.826, 19.446)
  line L699 (4.826, 24.526) -> (5.334, 24.526)
  line L700 (5.334, 19.446) -> (5.334, 19.954)
  line L701 (7.874, 17.414) -> (7.366, 17.414)
  line L702 (5.334, 29.606) -> (5.334, 30.114)
  line L703 (7.366, 24.526) -> (7.874, 24.526)
  line L704 (7.366, 14.874) -> (7.366, 14.366)
  line L705 (5.334, 24.526) -> (5.334, 25.034)
  line L706 (7.366, 14.366) -> (7.874, 14.366)
  line L707 (7.366, 25.034) -> (7.366, 24.526)
  line L708 (5.334, 27.574) -> (4.826, 27.574)
  line L709 (7.366, 19.954) -> (7.366, 19.446)
  line L710 (28.27, 15.705) -> (28.27, 11.895)
  line L711 (33.02, 53.975) -> (32.385, 53.975)
  arc A47 (38.5, 55.7) -> (41.5, 55.7) centre (40, 56.5) ccw
  line L712 (28.905, 11.26) -> (30.175, 11.26)
  line L713 (26.365, 11.26) -> (27.635, 11.26)
  line L714 (7.874, 22.494) -> (7.366, 22.494)
  line L715 (5.334, 14.874) -> (4.826, 14.874)
  line L716 (25.73, 11.895) -> (26.365, 11.26)
  line L717 (32.385, 53.975) -> (32.385, 53.34)
  line L718 (5.334, 14.366) -> (5.334, 14.874)
  line L719 (4.826, 17.414) -> (4.826, 16.906)
  line L720 (7.874, 14.874) -> (7.366, 14.874)
  line L721 (7.366, 17.414) -> (7.366, 16.906)
  line L722 (7.366, 16.906) -> (7.874, 16.906)
  line L723 (7.874, 16.906) -> (7.874, 17.414)
  line L724 (23.825, 16.34) -> (25.095, 16.34)
  line L725 (30.0038, 56.0388) -> (30.0038, 58.5787)
  line L726 (28.905, 16.34) -> (30.175, 16.34)
  line L727 (37.3062, 45.8788) -> (34.7662, 45.8788)
  line L728 (34.7662, 45.8788) -> (34.7662, 38.2587)
  line L729 (37.3062, 38.2587) -> (37.3062, 45.8788)
  line L730 (23.19, 11.895) -> (23.19, 11.26)
  line L731 (32.385, 50.8) -> (33.02, 51.435)
  line L732 (37.3062, 38.2587) -> (39.8463, 38.2587)
  line L733 (38.5763, 45.8788) -> (38.5763, 46.6408)
  arc A48 (41.5, 57.3) -> (38.5, 57.3) centre (40, 56.5) ccw
  line L734 (25.095, 16.34) -> (25.73, 15.705)
  line L735 (36.0363, 38.2587) -> (36.0363, 37.4967)
  line L736 (34.29, 48.895) -> (33.02, 48.895)
  line L737 (23.19, 11.895) -> (23.19, 15.705)
  line L738 (27.635, 16.34) -> (28.27, 15.705)
  line L739 (30.175, 16.34) -> (30.81, 15.705)
  line L740 (34.925, 50.8) -> (34.925, 49.53)
  line L741 (28.27, 11.895) -> (28.905, 11.26)
  line L742 (32.385, 49.53) -> (32.385, 50.8)
  line L743 (30.175, 11.26) -> (30.81, 11.895)
  line L744 (34.925, 52.07) -> (34.29, 51.435)
  line L745 (23.19, 11.26) -> (25.095, 11.26)
  line L746 (34.7662, 38.2587) -> (34.7662, 45.8788)
  line L747 (43.6563, 38.2587) -> (43.6563, 37.4967)
  line L748 (41.1163, 38.2587) -> (41.1163, 37.4967)
  line L749 (39.8463, 38.2587) -> (42.3863, 38.2587)
  arc A49 (38.5, 55.7) -> (41.5, 55.7) centre (40, 56.5) ccw
  line L750 (34.29, 53.975) -> (33.02, 53.975)
  line L751 (34.29, 51.435) -> (34.925, 50.8)
  line L752 (44.9263, 45.8788) -> (42.3863, 45.8788)
  line L753 (28.27, 15.705) -> (28.905, 16.34)
  line L754 (22.3838, 57.3088) -> (21.6218, 57.3088)
  line L755 (42.3863, 38.2587) -> (42.3863, 45.8788)
  line L756 (38.5763, 38.2587) -> (38.5763, 37.4967)
  line L757 (39.8463, 45.8788) -> (39.8463, 38.2587)
  line L758 (43.6563, 45.8788) -> (43.6563, 46.6408)
  line L759 (34.29, 51.435) -> (33.02, 51.435)
  line L760 (25.73, 15.705) -> (25.73, 11.895)
  line L761 (42.3863, 45.8788) -> (42.3863, 38.2587)
  line L762 (23.19, 15.705) -> (23.825, 16.34)
  line L763 (37.3062, 45.8788) -> (37.3062, 38.2587)
  line L764 (34.925, 49.53) -> (34.29, 48.895)
  line L765 (42.3863, 38.2587) -> (44.9263, 38.2587)
  line L766 (25.73, 15.705) -> (26.365, 16.34)
  line L767 (27.635, 11.26) -> (28.27, 11.895)
  line L768 (36.0363, 45.8788) -> (36.0363, 46.6408)
  line L769 (34.925, 53.34) -> (34.29, 53.975)
  line L770 (30.81, 15.705) -> (30.81, 11.895)
  line L771 (25.095, 11.26) -> (25.73, 11.895)
  line L772 (33.02, 51.435) -> (32.385, 52.07)
  arc A50 (41.5, 57.3) -> (38.5, 57.3) centre (40, 56.5) ccw
  line L773 (34.7662, 38.2587) -> (37.3062, 38.2587)
  line L774 (39.8463, 38.2587) -> (39.8463, 45.8788)
  line L775 (26.365, 16.34) -> (27.635, 16.34)
  line L776 (33.02, 48.895) -> (32.385, 49.53)
  line L777 (41.1163, 45.8788) -> (41.1163, 46.6408)
  line L778 (32.385, 52.07) -> (32.385, 53.34)
  line L779 (39.8463, 45.8788) -> (37.3062, 45.8788)
  line L780 (30.0038, 58.5787) -> (22.3838, 58.5787)
  circle A51 centre (23, 65) radius 1.75
  line L781 (42.4498, 33.9408) -> (39.1478, 33.9408)
  line L782 (44.9263, 38.2587) -> (44.9263, 45.8788)
  line L783 (42.4498, 22.7647) -> (39.1478, 22.7647)
  line L784 (42.7037, 25.0508) -> (42.7037, 23.5267)
  line L785 (38.8938, 28.6068) -> (38.8938, 30.1308)
  arc A52 (20.55, 66.75) -> (20.5, 67.5) centre (20.8502, 67.1467) ccw
  line L786 (32.2263, 38.2587) -> (34.7662, 38.2587)
  line L787 (38.8938, 31.1468) -> (38.8938, 32.6707)
  line L788 (39.1478, 22.2568) -> (42.4498, 22.2568)
  line L789 (35.8458, 33.9408) -> (35.8458, 22.2568)
  line L790 (42.7037, 30.1308) -> (38.8938, 30.1308)
  line L791 (38.8938, 26.0668) -> (38.8938, 27.5907)
  line L792 (42.7037, 30.1308) -> (42.7037, 28.6068)
  line L793 (38.8938, 23.5267) -> (38.8938, 25.0508)
  line L794 (38.8938, 23.5267) -> (42.7037, 23.5267)
  line L795 (42.7037, 27.5907) -> (42.7037, 26.0668)
  line L796 (22.3838, 56.0388) -> (30.0038, 56.0388)
  circle A53 centre (23, 65) radius 1.4
  line L797 (42.3863, 45.8788) -> (39.8463, 45.8788)
  line L798 (39.1478, 33.9408) -> (39.1478, 33.4327)
  line L799 (30.0038, 57.3088) -> (30.7658, 57.3088)
  line L800 (26, 66.45) -> (26, 63.6)
  line L801 (42.4498, 22.2568) -> (42.4498, 22.7647)
  line L802 (39.1478, 33.4327) -> (42.4498, 33.4327)
  line L803 (39.1478, 22.7647) -> (39.1478, 22.2568)
  line L804 (38.8938, 28.6068) -> (42.7037, 28.6068)
  line L805 (42.4498, 22.2568) -> (45.7518, 22.2568)
  line L806 (40.7988, 23.7808) -> (39.1478, 23.7808)
  line L807 (42.7037, 32.6707) -> (38.8938, 32.6707)
  line L808 (33.4963, 38.2587) -> (33.4963, 37.4967)
  line L809 (40.7988, 24.7968) -> (39.1478, 24.7968)
  arc A54 (25.45, 67.55) -> (25.5, 66.8) centre (25.1498, 67.1533) ccw
  line L810 (34.7662, 45.8788) -> (32.2263, 45.8788)
  line L811 (33.4963, 45.8788) -> (33.4963, 46.6408)
  line L812 (25.4, 62) -> (20.25, 62)
  line L813 (20.25, 68) -> (25.75, 68)
  line L814 (39.1478, 33.9408) -> (35.8458, 33.9408)
  line L815 (40.7988, 29.8768) -> (39.1478, 29.8768)
  line L816 (32.2263, 45.8788) -> (32.2263, 38.2587)
  line L817 (45.7518, 22.2568) -> (45.7518, 33.9408)
  line L818 (22.3838, 58.5787) -> (22.3838, 56.0388)
  line L819 (42.4498, 33.4327) -> (42.4498, 33.9408)
  line L820 (35.8458, 22.2568) -> (39.1478, 22.2568)
  line L821 (40.7988, 26.3208) -> (39.1478, 26.3208)
  line L822 (42.7037, 32.6707) -> (42.7037, 31.1468)
  arc A55 (25.45, 63.25) -> (25.45, 62.45) centre (25.15, 62.85) ccw
  line L823 (42.7037, 27.5907) -> (38.8938, 27.5907)
  line L824 (45.7518, 33.9408) -> (42.4498, 33.9408)
  arc A56 (20.55, 62.45) -> (20.5, 63.2) centre (20.8502, 62.8467) ccw
  line L825 (40.7988, 28.8608) -> (39.1478, 28.8608)
  line L826 (38.8938, 31.1468) -> (42.7037, 31.1468)
  line L827 (40.7988, 32.4168) -> (39.1478, 32.4168)
  line L828 (40.7988, 31.4008) -> (39.1478, 31.4008)
  line L829 (38.8938, 26.0668) -> (42.7037, 26.0668)
  line L830 (40.7988, 27.3368) -> (39.1478, 27.3368)
  line L831 (20, 63.55) -> (20, 66.45)
  line L832 (40.7988, 27.3368) -> (40.4178, 27.3368)
  line L833 (39.5288, 32.4168) -> (39.1478, 32.4168)
  line L834 (39.5288, 24.7968) -> (39.1478, 24.7968)
  line L835 (40.1638, 27.3368) -> (39.7828, 27.3368)
  line L836 (39.1478, 24.7968) -> (39.1478, 23.7808)
  line L837 (40.7988, 26.3208) -> (40.7988, 27.3368)
  line L838 (40.4178, 28.8608) -> (40.7988, 28.8608)
  line L839 (40.1638, 26.3208) -> (40.1638, 27.3368)
  line L840 (41.7, 53.3) -> (40.8, 53.3)
  line L841 (40.4178, 27.3368) -> (40.4178, 26.3208)
  line L842 (39.7828, 32.4168) -> (39.7828, 31.4008)
  line L843 (40.7988, 23.7808) -> (40.7988, 24.7968)
  line L844 (40.1638, 31.4008) -> (40.1638, 32.4168)
  line L845 (39.1478, 31.4008) -> (39.5288, 31.4008)
  line L846 (40.7988, 28.8608) -> (40.7988, 29.8768)
  line L847 (42.7037, 25.0508) -> (38.8938, 25.0508)
  line L848 (40.7988, 29.8768) -> (40.4178, 29.8768)
  line L849 (40.3, 14.5) -> (40.3, 13.1)
  line L850 (44.5, 49.7) -> (43.3, 49.7)
  line L851 (39.5288, 23.7808) -> (39.5288, 24.7968)
  line L852 (40.1638, 23.7808) -> (40.1638, 24.7968)
  line L853 (39.1478, 29.8768) -> (39.1478, 28.8608)
  line L854 (39.7828, 29.8768) -> (39.7828, 28.8608)
  line L855 (40.1638, 32.4168) -> (39.7828, 32.4168)
  line L856 (39.5288, 29.8768) -> (39.1478, 29.8768)
  line L857 (35.5, 12) -> (36.7, 12)
  line L858 (39.7828, 27.3368) -> (39.7828, 26.3208)
  line L859 (40.4178, 26.3208) -> (40.7988, 26.3208)
  line L860 (39.7828, 31.4008) -> (40.1638, 31.4008)
  line L861 (40.4178, 32.4168) -> (40.4178, 31.4008)
  line L862 (38.3, 52.2) -> (38.3, 50.8)
  line L863 (40.1638, 28.8608) -> (40.1638, 29.8768)
  line L864 (39.7828, 24.7968) -> (39.7828, 23.7808)
  line L865 (40.1638, 29.8768) -> (39.7828, 29.8768)
  line L866 (39.5288, 28.8608) -> (39.5288, 29.8768)
  line L867 (40.7988, 32.4168) -> (40.4178, 32.4168)
  line L868 (39.5288, 27.3368) -> (39.1478, 27.3368)
  line L869 (39.1478, 32.4168) -> (39.1478, 31.4008)
  line L870 (40.7988, 24.7968) -> (40.4178, 24.7968)
  line L871 (39.1478, 26.3208) -> (39.5288, 26.3208)
  line L872 (39.5288, 31.4008) -> (39.5288, 32.4168)
  line L873 (39.7828, 28.8608) -> (40.1638, 28.8608)
  line L874 (44.5, 49.7) -> (44.5, 53.3)
  line L875 (35.5, 15.6) -> (35.5, 12)
  line L876 (40.7988, 31.4008) -> (40.7988, 32.4168)
  line L877 (40.4178, 31.4008) -> (40.7988, 31.4008)
  line L878 (35.5, 15.6) -> (36.7, 15.6)
  line L879 (40.4178, 23.7808) -> (40.7988, 23.7808)
  line L880 (39.5288, 26.3208) -> (39.5288, 27.3368)
  line L881 (39.1478, 27.3368) -> (39.1478, 26.3208)
  line L882 (39.1478, 28.8608) -> (39.5288, 28.8608)
  line L883 (39.7828, 26.3208) -> (40.1638, 26.3208)
  line L884 (40.4178, 24.7968) -> (40.4178, 23.7808)
  line L885 (40.4178, 29.8768) -> (40.4178, 28.8608)
  line L886 (39.1478, 23.7808) -> (39.5288, 23.7808)
  line L887 (39.7828, 23.7808) -> (40.1638, 23.7808)
  line L888 (40.1638, 24.7968) -> (39.7828, 24.7968)
  line L889 (41.7, 50.8) -> (41.7, 52.2)
  line L890 (38.3, 50.8) -> (41.7, 50.8)
  line L891 (35.4, 53.3) -> (36.7, 53.3)
  line L892 (38.3, 14.5) -> (38.3, 13.1)
  line L893 (38.3, 50.8) -> (39.7, 50.8)
  line L894 (38.3, 52.2) -> (38.3, 50.8)
  line L895 (38.3, 13.1) -> (41.7, 13.1)
  line L896 (41.7, 52.2) -> (38.3, 52.2)
  line L897 (35.4, 49.7) -> (36.7, 49.7)
  line L898 (39.7, 52.2) -> (38.3, 52.2)
  line L899 (38.3, 12) -> (39.2, 12)
  line L900 (44.6, 12) -> (44.6, 15.6)
  line L901 (40.8, 12) -> (41.7, 12)
  line L902 (41.7, 14.5) -> (40.3, 14.5)
  line L903 (39.2, 49.7) -> (38.3, 49.7)
  line L904 (40.3, 13.1) -> (41.7, 13.1)
  line L905 (41.7, 14.5) -> (38.3, 14.5)
  line L906 (44.5, 53.3) -> (43.3, 53.3)
  line L907 (41.7, 49.7) -> (40.8, 49.7)
  line L908 (41.7, 13.1) -> (41.7, 14.5)
  line L909 (40.8, 15.6) -> (41.7, 15.6)
  line L910 (35.4, 53.3) -> (35.4, 49.7)
  line L911 (44.6, 15.6) -> (43.3, 15.6)
  line L912 (44.6, 12) -> (43.3, 12)
  line L913 (41.7, 13.1) -> (41.7, 14.5)
  line L914 (38.3, 15.6) -> (39.2, 15.6)
  line L915 (39.7, 50.8) -> (39.7, 52.2)
  line L916 (39.2, 53.3) -> (38.3, 53.3)
  line L917 (26.746, 12.784) -> (26.746, 12.276)
  arc A57 (20.5, 63.2) -> (20.55, 62.45) centre (20.8502, 62.8467) ccw
  line L918 (38.5, 55.7) -> (38.5, 57.3)
  line L919 (29.286, 15.324) -> (29.286, 14.816)
  line L920 (20.25, 62) -> (20.2, 62)
  arc A58 (20, 62.2) -> (20.2, 62) centre (20.2, 62.2) ccw
  line L921 (26, 66.9) -> (26.5, 66.9)
  circle A59 centre (40, 56.5) radius 1.5
  line L922 (27.254, 12.784) -> (26.746, 12.784)
  line L923 (20, 66.9) -> (20, 67.6)
  line L924 (29.286, 12.276) -> (29.794, 12.276)
  line L925 (27.254, 12.276) -> (27.254, 12.784)
  line L926 (29.794, 12.784) -> (29.286, 12.784)
  line L927 (26.746, 15.324) -> (26.746, 14.816)
  line L928 (29.286, 14.816) -> (29.794, 14.816)
  line L929 (29.794, 14.816) -> (29.794, 15.324)
  line L930 (29.794, 15.324) -> (29.286, 15.324)
  line L931 (26, 63.6) -> (26, 62.2)
  line L932 (26, 67.6) -> (26, 66.9)
  arc A60 (41.5, 55.7) -> (41.5, 57.3) centre (40, 56.5) ccw
  line L933 (19.5, 62.4) -> (20, 62.4)
  line L934 (19.5, 63.1) -> (19.5, 62.4)
  line L935 (29.286, 12.784) -> (29.286, 12.276)
  line L936 (26, 67.8) -> (26, 66.45)
  arc A61 (25.5, 66.8) -> (25.45, 67.55) centre (25.1498, 67.1533) ccw
  line L937 (20, 67.6) -> (19.5, 67.6)
  line L938 (26.5, 67.6) -> (26, 67.6)
  line L939 (26.5, 66.9) -> (26.5, 67.6)
  line L940 (29.794, 12.276) -> (29.794, 12.784)
  arc A62 (20.5, 67.5) -> (20.55, 66.75) centre (20.8502, 67.1467) ccw
  line L941 (20, 62.4) -> (20, 63.1)
  line L942 (26.746, 12.276) -> (27.254, 12.276)
  line L943 (20.2, 68) -> (20.25, 68)
  line L944 (26.5, 62.4) -> (26.5, 63.1)
  line L945 (20, 66.45) -> (20, 67.8)
  arc A63 (25.45, 62.45) -> (25.45, 63.25) centre (25.15, 62.85) ccw
  arc A64 (25.8, 62) -> (26, 62.2) centre (25.8, 62.2) ccw